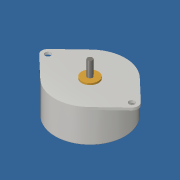
# Autodesk Inventor part: Stepper_42mm
Saved by Autodesk Inventor 2016 (Build 200138000, 138)
## iProperties
Created: 2016-03-10
Part Number: Stepper_42mm
Material: Aluminium 6061
Document SubType Name: Modeling
Designer: 4ndreas
Density: 2.7 g/cm^3
Appearance: Aluminium - flach
Mass: 75.873 g
Surface Area: 58.9763 cm^2
Volume: 28.1011 cm^3
Author: 4ndreas
Autodesk Inventor part; units mm, degrees
ref_plane "YZ Plane" through (0, 0, 0) normal (1, 0, 0) x (0, 1, 0)
ref_plane "XZ Plane" through (0, 0, 0) normal (0, 1, 0) x (-1, 0, 0)
sketch "Skizze1" plane through (0, 0, 0) normal (0, 0, 1) x (1, 0, 0)
  circle A0 centre (0, 0) radius 21
  circle A1 centre (0, 0) radius 25 construction
  circle A2 centre (-25, 0) radius 1.75
  circle A3 centre (25, 0) radius 1.75
  arc A4 (-27.5875, 2.7143) -> (-27.5875, -2.7143) centre (-25, 0) ccw
  arc A5 (27.5875, -2.7143) -> (27.5875, 2.7143) centre (25, 0) ccw
  line L0 (-27.5875, 2.7143) -> (-14.49, 15.2)
  line L1 (-27.5875, -2.7143) -> (-14.49, -15.2)
  line L2 (14.49, -15.2) -> (27.5875, -2.7143)
  line L3 (14.49, 15.2) -> (27.5875, 2.7143)
  line L4 (-25, 0) -> (25, 0) construction
  circle A6 centre (0, 0) radius 1.5
  dimension "d0" = 42
  dimension "d1" = 3.5
  dimension "d2" = 50
  dimension "d3" = 2
  dimension "d8" = 3
  constraints: 10 end point, 10 point on circle, 8 tangent, 7 centre point, 5 coincident, 1 equal length, 1 equal radius, 1 horizontal, 1 midpoint
  measures "d0" diameter of A0
  measures "d1" diameter of A3
  measures "d2" diameter of A1
  measures "d3" radial gap between concentric circles of A3 A5
  measures "d8" diameter of A6
extrude "Extrusion1" add sketch "Skizze1" against normal blind 1.5 contours A0 | A0 L3 A5 L2 | A0 L1 A4 L0 | A6
extrude "Extrusion2" add sketch "Skizze1" against normal blind 20 contours A0 | A6
extrude "Extrusion3" add sketch "Skizze1" along normal blind 10 contours A6
sketch "Skizze2" plane through (0, 0, 0) normal (0, 0, 1) x (1, 0, 0)
  circle A0 centre (0, 0) radius 5
  dimension "d11" = 10
  constraints: 1 centre point, 1 coincident
  measures "d11" diameter of A0
extrude "Extrusion4" add sketch "Skizze2" along normal blind 1
ref_plane "Arbeitsebene1" through (0, 0, 0) normal (0, 0, 1) x (1, 0, 0)
fillet "Rundung1" radius 1 1 edges at (14.49, 15.2, -20)
sketch "Skizze3" plane through (0, 0, -20) normal (0, 0, -1) x (-1, 0, 0)
  circle A0 centre (0, 0) radius 21
  line L0 (-18.963, -9.0226) -> (-8.1058, -19.3726)
  line L1 (-8.1058, -19.3726) -> (-15.0058, -26.6106)
  line L2 (-15.0058, -26.6106) -> (-25.863, -16.2606)
  line L3 (-25.863, -16.2606) -> (-18.963, -9.0226)
  line L4 (0, 0) -> (-20.4344, -21.4356) construction
  circle A1 centre (0, 0) radius 21 construction
  arc A2 (-14.49, 15.2) -> (-14.49, -15.2) centre (0, 0) ccw construction
  line L5 (-14.49, 15.2) -> (-27.5875, 2.7143) construction
  arc A3 (-27.5875, 2.7143) -> (-27.5875, -2.7143) centre (-25, 0) ccw construction
  line L6 (-27.5875, -2.7143) -> (-14.49, -15.2) construction
  circle A4 centre (-25, 0) radius 1.75 construction
  point P0 (-13.5344, -14.1976)
  dimension "d15" = 15
  dimension "d16" = 10
  constraints: 14 end point, 4 point on circle, 3 centre point, 3 parallel, 2 midpoint, 1 perpendicular, 1 point on line, 6 other
  measures "d15" distance between parallel lines of L1 L3
  measures "d16" distance between parallel lines of L2 L0
